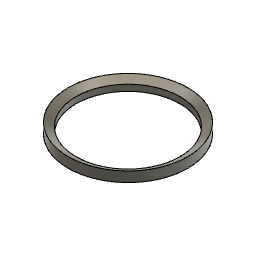
Wheel Spacer (Autodesk Fusion 360 design; units mm, degrees)
Autodesk Fusion 360 part; units mm, degrees
sketch "Sketch1" plane through (0, 0, 0) normal (0, 0, 1) x (1, 0, 0)
  line L0 (0, 0) -> (7.5, 0)
  line L1 (0, 0) -> (0, 3)
  line L2 (7.5, 0) -> (7.5, 6.75)
  line L3 (0, 3) -> (7.5, 6.75)
  dimension "d1" = 7.5
  dimension "d2" = 3
  dimension "d3" = 6.75
  constraint coincident L0.start L1.start
  constraint horizontal L0
  constraint perpendicular L0 L1
  constraint perpendicular L0 L2
  measures "d1" distance of L0.start L0.end
  measures "d2" distance of L0.start L1.end
  measures "d3" distance of L0.end L2.end
sketch "Sketch2" plane through (0, 0, 0) normal (0, 1, 0) x (1, 0, 0)
  line L0 (0, 0) -> (-50.25, 0)
  circle A0 centre (-50.25, 0) radius 2.5
  dimension "d4" = 50.25
  dimension "d6" = 5
  constraint coincident L0.start origin
  constraint horizontal L0
  constraint coincident L0.end A0.centre
  measures "d4" distance of L0.start L0.end
  measures "d6" diameter of A0
extrude "Extrude1" add sketch "Sketch2" along normal blind 100 makes body 1
revolve "Revolve1" add sketch "Sketch1" angle 360 about axis through (-50.25, 0, 0) along (0, -1, 0) separate body makes body 2
delete_body "RemoveBody1" bodies 1
extrude "Extrude2" add 1 faces at (4.5979, 0, -5.3655) along direction (0, -1, 0) blind 3 on bodies 2 bodies 2
equation "d3 = 3.75 mm + 3 mm"
equation "d4 = ( 100.5 / 2 ) * 1 mm"
